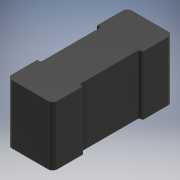
# Autodesk Inventor part: battery
Saved by Autodesk Inventor 2018 (Build 220112000, 112)
## iProperties
Created: 2018-01-18
Part Number: battery
Material: Generic
Document SubType Name: Modeling
Designer: Justin
Density: 1 g/cm^3
Appearance: Default
Author: Justin
Autodesk Inventor part; units mm, degrees
ref_plane "YZ Plane" through (0, 0, 0) normal (1, 0, 0) x (0, 1, 0)
ref_plane "XZ Plane" through (0, 0, 0) normal (0, 1, 0) x (-1, 0, 0)
ref_plane "XY Plane" through (0, 0, 0) normal (0, 0, 1) x (1, 0, 0)
sketch "Sketch1" plane through (0, 0, 0) normal (1, 0, 0) x (0, 1, 0)
  line L0 (130, 85.25) -> (-130, 85.25)
  line L1 (-130, 85.25) -> (-130, -85.25)
  line L2 (-130, -85.25) -> (130, -85.25)
  line L3 (130, -85.25) -> (130, 85.25)
  point P0 (0, 0)
  dimension "d0" = 170.5
  dimension "d1" = 260
  dimension "d2" = 85.25
  dimension "d3" = 130
  constraints: 8 end point, 2 parallel, 1 horizontal, 1 perpendicular
  measures "d0" distance between parallel lines of L2 L0
  measures "d1" distance between parallel lines of L1 L3
  measures "d2" distance from line of point (0, 0) L0
  measures "d3" distance from line of L1 point (0, 0)
extrude "Extrusion1" add sketch "Sketch1" against normal blind 197
sketch "Sketch2" plane through (0, -130, 85.25) normal (0, 0, 1) x (1, 0, 0)
  line L0 (-15, 130) -> (-15, 195)
  line L1 (-15, 195) -> (0, 195)
  line L2 (-15, 130) -> (-15, 65)
  line L3 (-15, 65) -> (0, 65)
  line L4 (0, 260) -> (-197, 260) projected
  line L5 (-98.5, 260) -> (-98.5, 0)
  line L6 (0, 0) -> (-197, 0) projected
  line L7 (-182, 130) -> (-182, 195)
  line L8 (-182, 195) -> (-197, 195)
  line L9 (-182, 130) -> (-182, 65)
  line L10 (-182, 65) -> (-197, 65)
  line L11 (-197, 195) -> (-197, 65)
  line L12 (0, 195) -> (0, 65)
  line L13 (0, 260) -> (0, 0) projected
  line L14 (-197, 0) -> (-197, 260) projected
  point P0 (0, 130)
  dimension "d8" = 65
  dimension "d9" = 65
  dimension "d10" = 15
  dimension "d11" = 0
  dimension "d12" = 65
  constraints: 22 end point, 5 symmetric about line, 2 midpoint, 1 collinear, 1 perpendicular, 1 vertical
  measures "d8" distance of L0.start L0.end
  measures "d9" distance of L0.start L2.end
  measures "d10" distance between parallel lines of L12 L0
  measures "d11" distance between parallel lines of L14 L11
  measures "d12" distance from line of point (0, 130) L1
extrude "Extrusion2" cut sketch "Sketch2" against normal blind 197 contours L0 L1 L12 L3 L2 | L8 L7 L9 L10 L11
scale "Scale1" factors (2, 4, 3) then translate (182, -195, 170.5) bodies 1
fillet "Fillet2" radius 40 4 edges at (182, -715, 170.5) (182, 325, 170.5) (-212, 325, 170.5) (-212, -715, 170.5)
fillet "Fillet3" radius 15 4 edges at (152, 65, 170.5) (-182, 65, 170.5) (-182, -455, 170.5) (152, -455, 170.5)
body "Solid1"
